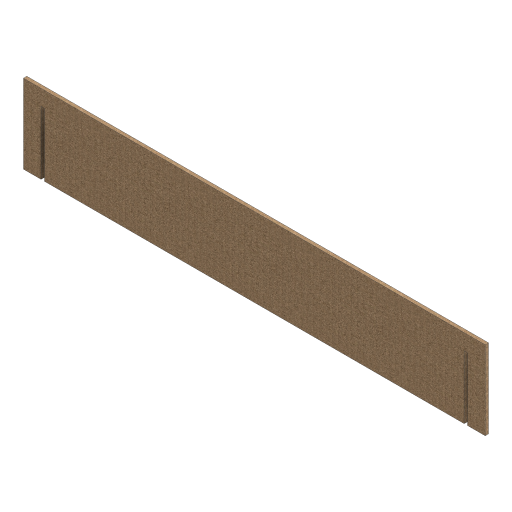
# Autodesk Inventor part: PARED_ESTRUCTURAL
Saved by Autodesk Inventor 2024.2 (Build 282272000, 272)
## iProperties
Created: 2024-07-19
Part Number: PARED_ESTRUCTURAL
Material: MDF Medium Density Fiberboard
Document SubType Name: Modeling
Designer: jrcer
Density: 0.8 g/cm^3
Appearance: Cardboard - Corrugated
Author: jrcer
Autodesk Inventor part; units mm, degrees
ref_plane "YZ Plane" through (0, 0, 0) normal (1, 0, 0) x (0, 1, 0)
ref_plane "XZ Plane" through (0, 0, 0) normal (0, 1, 0) x (-1, 0, 0)
ref_plane "XY Plane" through (0, 0, 0) normal (0, 0, 1) x (1, 0, 0)
sketch "Sketch1" plane through (0, 0, 0) normal (0, 0, 1) x (1, 0, 0)
  line L0 (0, 0) -> (440, 0)
  line L1 (440, 0) -> (440, 75.1)
  line L2 (440, 75.1) -> (0, 75.1)
  line L3 (0, 75.1) -> (0, 0)
  line L4 (16.8, 60.1) -> (20, 60.1)
  line L5 (20, 60.1) -> (20, 0)
  line L6 (20, 0) -> (16.8, 0)
  line L7 (16.8, 0) -> (16.8, 60.1)
  line L8 (220, 75.1) -> (220, 0) construction
  line L9 (423.2, 60.1) -> (420, 60.1)
  line L10 (420, 60.1) -> (420, 0)
  line L11 (420, 0) -> (423.2, 0)
  line L12 (423.2, 0) -> (423.2, 60.1)
  point P0 (420, 0)
  dimension "d0" = 440
  dimension "d1" = 75.1
  dimension "d2" = 200
  dimension "d3" = 3.2
  dimension "d4" = 15
  constraints: 26 end point, 4 parallel, 4 symmetric about line, 2 horizontal, 2 midpoint, 2 perpendicular, 1 point on line
  measures "d0" distance of L2.end L1.end
  measures "d1" distance of L1.end L0.end
  measures "d2" distance between parallel lines of L5 L8
  measures "d3" distance between parallel lines of L7 L5
  measures "d4" distance between parallel lines of L4 L2
extrude "Extrusion1" add sketch "Sketch1" along normal blind 3.2 contours L3 L2 L1 L0 L12 L9 L10 L5 L4 L7
body "Solid1"
